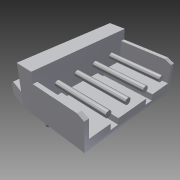
# Autodesk Inventor part: 2mmWireBoardConn
Saved by Autodesk Inventor 2014 (Build 180170000, 170)
## iProperties
Created: 2015-11-06
Part Number: 2mmWireBoardConn
Material: Generic
Document SubType Name: Modeling
Designer: Owner
Density: 1 g/cm^3
Appearance: Default
Author: Owner
Autodesk Inventor part; units mm, degrees
ref_plane "YZ Plane" through (0, 0, 0) normal (1, 0, 0) x (0, 1, 0)
ref_plane "XZ Plane" through (0, 0, 0) normal (0, 1, 0) x (-1, 0, 0)
ref_plane "XY Plane" through (0, 0, 0) normal (0, 0, 1) x (1, 0, 0)
sketch "Sketch1" plane through (0, 0, 0) normal (0, 0, 1) x (1, 0, 0)
  line L0 (-0.7045, 1.4865) -> (6.0955, 1.4865)
  line L1 (6.0955, 1.4865) -> (6.0955, -2.5135)
  line L2 (6.0955, -2.5135) -> (-0.7045, -2.5135)
  line L3 (-0.7045, -2.5135) -> (-0.7045, 1.4865)
  line L4 (0.9955, 1.4865) -> (0.9955, 0.4865)
  line L5 (0.9955, 0.4865) -> (5.4766, 0.4865)
  line L6 (5.4766, 0.4865) -> (6.0955, 0.2015)
  line L7 (-0.7045, -1.0135) -> (-2.2782, -1.0135)
  line L8 (-2.2782, -1.0135) -> (-2.7045, -1.3759)
  line L9 (-2.7045, -1.3759) -> (-2.7045, -2.5135)
  line L10 (-2.7045, -2.5135) -> (-0.7045, -2.5135)
  point P0 (0, 0)
  dimension "d0" = 6.8
  dimension "d1" = 4
  dimension "d2" = 1.7
  dimension "d3" = 1
  dimension "d4" = 8.8
  dimension "d5" = 1.5
  constraints: 22 end point, 5 parallel, 3 perpendicular, 3 point on line, 1 horizontal
  measures "d0" distance of L1.end L2.end
  measures "d1" distance of L0.end L1.end
  measures "d2" distance between parallel lines of L3 L4
  measures "d3" distance between parallel lines of L5 L0
  measures "d4" distance between parallel lines of L1 L9
  measures "d5" distance between parallel lines of L10 L7
extrude "Extrusion1" add sketch "Sketch1" along normal blind 9.8 contours L0 L4 L5 L6 L1 L2 L3 | L3 L10 L9 L8 L7
sketch "Sketch2" plane through (0.9955, 0.4865, 0) normal (0, 1, 0) x (1, 0, 0)
  line L0 (0, 0) -> (0, -9.8) projected
  line L1 (4.4812, -9.8) -> (0, -9.8) projected
  line L2 (6, -0.4) -> (0, -0.4)
  line L3 (0, -0.4) -> (0, -9.4)
  line L4 (0, -9.4) -> (6, -9.4)
  line L5 (6, -9.4) -> (6, -0.4)
  point P0 (-0.9955, 0)
  dimension "d8" = 9
  dimension "d9" = 0.4
  dimension "d10" = 6
  constraints: 8 end point, 2 parallel, 1 horizontal, 1 perpendicular, 1 point on line
  measures "d8" distance of L4.end L2.start
  measures "d9" distance between parallel lines of L1 L4
  measures "d10" distance between parallel lines of L0 L5
extrude "Extrusion2" cut sketch "Sketch2" against normal blind 2
sketch "Sketch3" plane through (0.9955, -1.5135, 0) normal (0, 1, 0) x (1, 0, 0)
  line L0 (0, -9.4) -> (0, -0.4) projected
  line L1 (0, -6.5) -> (5.6296, -6.5)
  line L2 (5.6296, -6.5) -> (5.6296, -7.3)
  line L3 (5.6296, -7.3) -> (0, -7.3)
  line L4 (0, -7.3) -> (0, -6.5)
  line L5 (0, -2.5) -> (5.6296, -2.5)
  line L6 (5.6296, -2.5) -> (5.6296, -3.3)
  line L7 (5.6296, -3.3) -> (0, -3.3)
  line L8 (0, -3.3) -> (0, -2.5)
  line L9 (4.4812, -9.8) -> (0, -9.8) projected
  point P0 (-0.9955, 0)
  dimension "d13" = 0.8
  dimension "d14" = 0.8
  dimension "d15" = 3.2
  dimension "d16" = 3.3
  constraints: 16 end point, 4 parallel, 2 horizontal, 2 perpendicular, 2 point on line
  measures "d13" distance of L5.end L6.end
  measures "d14" distance of L1.end L2.end
  measures "d15" distance between parallel lines of L1 L7
  measures "d16" distance between parallel lines of L9 L1
extrude "Extrusion3" cut sketch "Sketch3" against normal blind 0.6
sketch "Sketch6" plane through (6.0955, -2.5135, 0) normal (1, 0, 0) x (0, 0, -1)
  line L0 (-3.3, 1) -> (-6.5, 1) projected
  line L1 (-7.3, 1) -> (-9.4, 1) projected
  line L2 (-9.8, 0) -> (-9.8, 2.715) projected
  line L3 (-0.4, 1) -> (-2.5, 1) projected
  circle A0 centre (-7.6, 2) radius 0.3
  circle A1 centre (-5.6, 2) radius 0.3
  circle A2 centre (-3.6, 2) radius 0.3
  circle A3 centre (-1.6, 2) radius 0.3
  point P0 (0, 2.5135)
  dimension "d21" = 2.2
  dimension "d22" = 2
  dimension "d23" = 2
  dimension "d24" = 2
  dimension "d25" = 1
  dimension "d26" = 1
  dimension "d27" = 1
  dimension "d28" = 1
  dimension "d29" = 0.6
  dimension "d30" = 0.6
  dimension "d31" = 0.6
  dimension "d32" = 0.6
  constraints: 4 centre point
  measures "d21" distance from line of L2 A0.centre
  measures "d22" distance of A1.centre A0.centre
  measures "d23" distance of A2.centre A1.centre
  measures "d24" distance of A3.centre A2.centre
  measures "d25" distance from line of L1 A0.centre
  measures "d26" distance from line of L0 A1.centre
  measures "d27" distance from line of L0 A2.centre
  measures "d28" distance from line of L3 A3.centre
  measures "d29" diameter of A0
  measures "d30" diameter of A1
  measures "d31" diameter of A2
  measures "d32" diameter of A3
extrude "Extrusion4" add sketch "Sketch6" against normal blind 7
sketch "Sketch8" plane through (-2.2782, -1.0135, 0) normal (0, 1, 0) x (1, 0, 0)
  line L0 (1.5737, 0) -> (0, 0) projected
  line L1 (1.5737, 0) -> (1.5737, -9.8) projected
  line L2 (1.5737, -9.8) -> (-2.262, -9.8)
  line L3 (-2.262, -9.8) -> (-2.2372, 0)
  line L4 (-2.2372, 0) -> (1.2362, 0)
  line L5 (-0.8777, -0.4503) -> (1.2362, 0)
  line L6 (-0.8777, -0.4503) -> (-0.8777, -0.7872)
  line L7 (-0.8777, -0.7872) -> (1.5737, -1.307)
  line L8 (1.5737, -1.307) -> (1.5737, -1.9292)
  line L9 (1.5737, -1.9292) -> (-0.9327, -2.463)
  line L10 (-0.9327, -2.463) -> (-0.9327, -2.783)
  line L11 (-0.9327, -2.783) -> (1.5737, -3.3145)
  line L12 (1.5737, -3.3145) -> (1.5737, -3.9081)
  line L13 (1.5737, -3.9081) -> (-1.0204, -4.4607)
  line L14 (-1.0204, -4.4607) -> (-1.0204, -4.7289)
  line L15 (-1.0204, -4.7289) -> (1.5737, -5.3179)
  line L16 (1.5737, -5.3179) -> (1.5737, -5.906)
  line L17 (1.5737, -5.906) -> (-0.9385, -6.4411)
  line L18 (-0.9385, -6.4411) -> (-0.9385, -6.767)
  line L19 (-0.9385, -6.767) -> (1.5737, -7.3035)
  line L20 (1.5737, -7.3035) -> (1.5737, -7.9182)
  line L21 (1.5737, -7.9182) -> (-1.0783, -8.4831)
  line L22 (-1.0783, -8.4831) -> (-1.0783, -9.2337)
  line L23 (-1.0783, -9.2337) -> (1.5737, -9.8)
  point P0 (2.2782, 0)
  constraints: 44 end point, 10 parallel, 1 horizontal, 1 perpendicular, 1 point on line, 9 other
extrude "Extrusion5" cut sketch "Sketch8" against normal through all contours L5 L6 L7 L1 L9 L10 L11 L13 L14 L15 L17 L18 L19 L21 L22 L23 L2 L3 L4 L0
sketch "Sketch9" plane through (6.0955, -2.5135, 0) normal (0, -1, 0) x (1, 0, 0)
  line L0 (-6.8, 5.906) -> (-6.8, 5.3179) projected
  line L1 (-6.8, 3.9081) -> (-6.8, 3.3145) projected
  line L2 (-6.8, 1.9292) -> (-6.8, 1.307) projected
  line L3 (-6.8, 7.9182) -> (-6.8, 7.3035) projected
  circle A0 centre (-6.8, 1.6113) radius 0.3
  circle A1 centre (-6.8, 7.6108) radius 0.3
  circle A2 centre (-6.8, 5.612) radius 0.3
  circle A3 centre (-6.8, 3.6113) radius 0.3
  point P0 (-6.0955, 0)
  dimension "d54" = 0.6
  dimension "d56" = 0.6
  dimension "d57" = 0.6
  dimension "d58" = 0.6
  dimension "d59" = 2
  constraints: 4 centre point, 3 midpoint, 1 point on line
  measures "d54" diameter of A0
  measures "d56" diameter of A1
  measures "d57" diameter of A2
  measures "d58" diameter of A3
  measures "d59" distance of A0.centre A3.centre
extrude "Extrusion6" add sketch "Sketch9" along normal blind 3.2 and the other way blind 2
body "Solid1"
